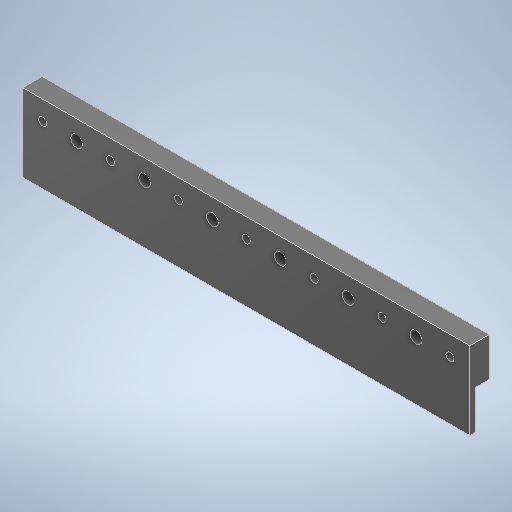
# Autodesk Inventor part: IR_Mount_Plate
Saved by Autodesk Inventor 2025.1 (Build 291241020, 241B)
## iProperties
Created: 2024-11-14
Part Number: IR_Mount_Plate
Material: PC/ABS Plastic
Document SubType Name: Modeling
Designer: leon-
Density: 1.1 g/cm^3
Appearance: Smooth - Black
Author: leon-
## iProperties of the stored document IR_Mount_Plate_3DPrint.ipt
Created: 2024-11-19
Part Number: IR_Mount_Plate_3DPrint
Material: Generic
Document SubType Name: Modeling
Designer: leon-
Density: 1 g/cm^3
Appearance: Default
Author: leon-
Autodesk Inventor part; units mm, degrees
ref_plane "YZ Plane" through (0, 0, 0) normal (1, 0, 0) x (0, 1, 0)
ref_plane "XZ Plane" through (0, 0, 0) normal (0, 1, 0) x (-1, 0, 0)
ref_plane "XY Plane" through (0, 0, 0) normal (0, 0, 1) x (1, 0, 0)
sketch "Sketch1" plane through (0, 0, 0) normal (0, 0, 1) x (1, 0, 0)
  line L0 (0, 0) -> (230, 0)
  line L1 (230, 0) -> (230, 20)
  line L2 (230, 20) -> (0, 20)
  line L3 (0, 20) -> (0, 0)
  dimension "d0" = 230
  dimension "d1" = 20
  constraints: 8 end point, 2 parallel, 1 horizontal, 1 perpendicular
  measures "d0" distance of L1.end L2.end
  measures "d1" distance of L0.end L1.end
extrude "Extrusion1" add sketch "Sketch1" along normal blind 3
sketch "Sketch2" plane through (0, 0, 3) normal (0, 0, -1) x (-1, 0, 0)
  line L0 (0, 0) -> (-230, 0) projected
  line L1 (-12.5251, -24.7625) -> (-37.9251, -24.7625) projected
  line L2 (-230, 20) -> (0, 20) projected
  point P0 (-10.225, 30)
  dimension "d62" = 10
  dimension "d73" = 10.225
  measures "d62" distance from line of L2 point (-10.225, 30)
  measures "d73" horizontal distance of L2.end point (-10.225, 30)
sketch "Sketch5" plane through (0, 0, 0) normal (-1, 0, 0) x (0, 0, 1)
  line L0 (0, 20) -> (3, 20) projected
  line L1 (3, 20) -> (-7, 20)
  line L2 (-7, 20) -> (-7, 40)
  line L3 (-7, 40) -> (3, 40)
  line L4 (3, 40) -> (3, 20)
  point P0 (0, 0)
  point P1 (3, 30)
  point P2 (1.5, 20)
  point P3 (0, 20)
  dimension "d31" = 10
  dimension "d32" = 20
  constraints: 8 end point, 2 midpoint, 2 parallel, 1 horizontal, 1 perpendicular
  measures "d31" distance from line of L2 point (3, 30)
  measures "d32" distance from line of point (1.5, 20) L3
extrude "Extrusion3" add sketch "Sketch5" against normal up to surface (230 mm away)
hole "Hole3" at (10.225, 30, 3) direction (0, 0, -1) diameter 4.1 depth 6
sketch "Sketch6" plane through (0, 0, 3) normal (0, 0, 1) x (1, 0, 0)
  line L0 (0, 0) -> (0, 40) projected
  line L1 (230, 0) -> (230, 40) projected
  line L2 (0, 40) -> (230, 40) projected
  point P0 (27.6875, 30)
  dimension "d35" = 27.6875
  dimension "d51" = 10
  measures "d35" distance from line of point (27.687, 30) L0
  measures "d51" distance from line of L2 point (27.687, 30)
hole "Hole2" at (27.6875, 30, 3) direction (0, 0, -1) diameter 6 end through all
pattern_linear "Rectangular Pattern2" count 6 spacing 34.925 along (1, 0, 0) of "Hole2"
pattern_linear "Rectangular Pattern3" count 7 spacing 34.925 along (1, 0, 0) of "Hole3"
sketch "Sketch7" plane through (0, 0, 0) normal (-1, 0, 0) x (0, 0, 1)
  line L0 (0, 0) -> (3, 0) projected
  line L1 (0, 0) -> (3.6796, 0)
  line L2 (3.6796, 0) -> (3.6796, 5)
  line L3 (3.6796, 5) -> (0, 5)
  line L4 (0, 5) -> (0, 0)
  dimension "d66" = 5
  constraints: 8 end point, 2 parallel, 1 horizontal, 1 perpendicular
  measures "d66" distance of L1.end L2.end
body "Solid1"
